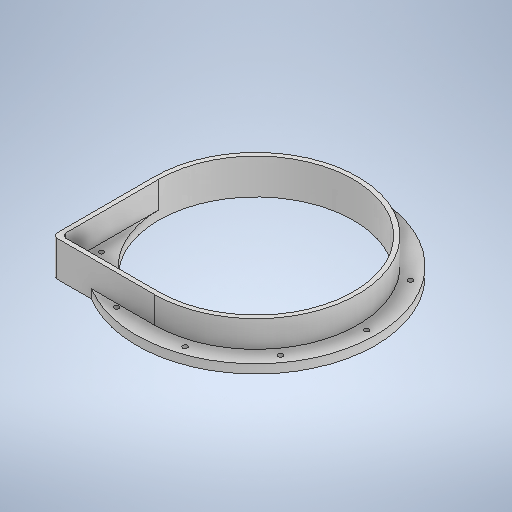
# Autodesk Inventor part: Cylinder Housing_base_3
Saved by Autodesk Inventor 2025 (Build 290162000, 162)
## iProperties
Created: 2025-09-30
Part Number: Cylinder Housing_base_3
Material: Generic
Document SubType Name: Modeling
Designer: mumin
Density: 1 g/cm^3
Appearance: Default
Author: mumin
Autodesk Inventor part; units mm, degrees
ref_plane "YZ Plane" through (0, 0, 0) normal (1, 0, 0) x (0, 1, 0)
ref_plane "XZ Plane" through (0, 0, 0) normal (0, 1, 0) x (-1, 0, 0)
ref_plane "XY Plane" through (0, 0, 0) normal (0, 0, 1) x (1, 0, 0)
sketch "Sketch1" plane through (0, 0, 0) normal (0, 1, 0) x (-1, 0, 0)
  circle A0 centre (0, 0) radius 135
  circle A1 centre (0, 0) radius 110
  dimension "d0" = 270
  dimension "d1" = 220
  constraints: 2 centre point, 2 coincident
  measures "d0" diameter of A0
  measures "d1" diameter of A1
extrude "Base" add sketch "Sketch1" along normal blind 10
sketch "Sketch2" plane through (0, 10, 0) normal (0, 1, 0) x (1, 0, 0)
  line L0 (-189, 0) -> (189, 0) projected
  point P0 (0, 0)
  point P1 (-125, 0)
  dimension "d11" = 125
  constraints: 1 point on line
  measures "d11" distance of point (0, 0) point (-125, 0)
hole "Cylinder Mount Holes" at (-125, 10, 0) direction (0, -1, 0) diameter 5.5 end through all
pattern_circular "Circular Pattern1" count 10 over 360 about axis through (0, 0, 0) along (0, 1, 0) of "Cylinder Mount Holes"
sketch "Sketch3" plane through (0, 10, 0) normal (0, 1, 0) x (1, 0, 0)
  arc A0 (0, -115) -> (-115, 0) centre (0, 0) ccw
  line L0 (-115, 0) -> (-110, 0)
  line L1 (0, -110) -> (0, -115)
  line L2 (0, -115) -> (-115, -115)
  line L3 (-115, -115) -> (-115, 0)
  arc A1 (0, -110) -> (-110, 0) centre (0, 0) ccw
  line L4 (0, -110) -> (-110, -110)
  line L5 (-110, -110) -> (-110, 0)
  dimension "d15" = 230
  dimension "d16" = 220
  constraints: 12 end point, 4 point on circle, 2 centre point, 2 parallel, 1 coincident, 1 horizontal, 1 perpendicular
  measures "d15" diameter of A0
  measures "d16" diameter of A1
extrude "Walls" add sketch "Sketch3" along normal blind 30 contours L1 A1 L0 A0 | L2 L3 L0 L5 L4 L1
sketch "Sketch4" plane through (0, 10, 0) normal (0, -1, 0) x (1, 0, 0)
  line L0 (-115, 70.7107) -> (-115, 115) projected
  line L1 (-115, 115) -> (-70.7107, 115) projected
  line L2 (-78.2624, 110) -> (-110, 110) projected
  line L3 (-110, 110) -> (-110, 78.2624) projected
  circle A0 centre (0, 0) radius 135 projected
extrude "Corner Fill" add sketch "Sketch4" along normal up to surface (10 mm away) contours L0 L1 A0 L2 L3 | L3 L2 A0
fillet "Fillet1" radius 5 2 edges at (-110, 25, 110) (-115, 20, 115)
sketch "Sketch6" plane through (0, 0, 0) normal (1, 0, 0) x (0, 1, 0)
  line L0 (0, -135) -> (0, 135) projected
  line L1 (0, 117.5) -> (2, 117.5)
  line L2 (2, 117.5) -> (2, 114.5)
  line L3 (2, 114.5) -> (0, 114.5)
  line L4 (0, 114.5) -> (0, 117.5)
  line L5 (-8, 0) -> (48, 0) projected
  point P0 (0, 0)
  point P1 (0, 115)
  point P2 (0, 70.7107)
  point P3 (0, 114.5)
  dimension "d26" = 2
  dimension "d27" = 3
  dimension "d28" = 117.5
  constraints: 8 end point, 2 parallel, 1 horizontal, 1 perpendicular, 1 point on line
  measures "d26" distance of L2.end L3.end
  measures "d27" distance of L1.end L2.end
  measures "d28" distance between parallel lines of L5 L1
revolve "Seal Groove" cut sketch "Sketch6" angle 360 about axis through (0, -10, 0) along (0, 1, 0)
body "Solid1"
